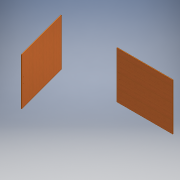
# Autodesk Inventor part: puerta_inf
Saved by Autodesk Inventor 2016 (Build 200138000, 138)
## iProperties
Created: 2015-11-25
Part Number: puerta_inf
Material: Generic
Document SubType Name: Modeling
Designer: Daniela
Density: 1 g/cm^3
Appearance: Glossy - Black
Author: Daniela
Autodesk Inventor part; units mm, degrees
ref_plane "YZ Plane" through (0, 0, 0) normal (1, 0, 0) x (0, 1, 0)
ref_plane "XZ Plane" through (0, 0, 0) normal (0, 1, 0) x (-1, 0, 0)
ref_plane "XY Plane" through (0, 0, 0) normal (0, 0, 1) x (1, 0, 0)
sketch "Sketch1" plane through (0, 0, 0) normal (0, 1, 0) x (-1, 0, 0)
  line L0 (0, 0) -> (-721.6667, 0)
  line L1 (-721.6667, 0) -> (-721.6667, 820)
  line L2 (-721.6667, 820) -> (0, 820)
  line L3 (0, 820) -> (0, 0)
  line L4 (0, 410) -> (-41, 410)
  line L5 (-41, 410) -> (-41, 460)
  line L6 (-41, 460) -> (-41, 360)
  circle A0 centre (-41, 460) radius 3
  circle A1 centre (-41, 360) radius 3
  dimension "ancho_m" = 721.6667
  dimension "h_inf" = 820
  dimension "d2" = 41
  dimension "d3" = 50
  dimension "d4" = 100
  dimension "d5" = 6
  dimension "d6" = 6
  constraints: 14 end point, 2 centre point, 2 coincident, 2 horizontal, 2 parallel, 2 perpendicular, 1 midpoint, 1 point on line
  measures "ancho_m" distance of L1.end L2.end
  measures "h_inf" distance of L0.end L1.end
  measures "d2" distance of L4.start L4.end
  measures "d3" distance of L4.end L5.end
  measures "d4" distance of L5.end L6.end
  measures "d5" diameter of A0
  measures "d6" diameter of A1
extrude "Extrusion1" add sketch "Sketch1" along normal blind 10
sketch "Boceto10" plane through (0, 0, 820) normal (0, 0, 1) x (1, 0, 0)
  line L0 (721.6667, 10) -> (0, 10) projected
  line L1 (0, 10) -> (-721.6667, 10)
  line L2 (-721.6667, 10) -> (-534.8856, -687.0765)
  line L3 (-721.6667, 10) -> (0, 10) construction
  line L4 (-534.8856, -687.0765) -> (-544.5448, -689.6647)
  line L5 (-544.5448, -689.6647) -> (-731.3259, 7.4118)
  line L6 (-731.3259, 7.4118) -> (-721.6667, 10)
  point P0 (0, 0)
  dimension "d49" = 721.6667
  dimension "d50" = 721.6667
  dimension "angulo" = 75
  dimension "d52" = 10
  dimension "d53" = 721.6667
  constraints: 12 end point, 2 horizontal, 2 perpendicular, 1 equal length
  measures "d49" distance of L0.end L1.end
  measures "d50" distance of L1.end L2.end
  measures "angulo" angle of L2 L3
  measures "d52" distance of L2.end L4.end
  measures "d53" distance of L4.end L5.end
extrude "Extrusión10" add sketch "Boceto10" against normal blind 820
sketch "Boceto11" plane through (-534.8856, -687.0765, 820) normal (0.9659258, 0.258819, 0) x (0, 0, -1)
  line L0 (0, 721.6667) -> (0, 0) projected
  line L1 (0, 0) -> (820, 0) projected
  line L2 (820, 721.6667) -> (820, 0) projected
  line L3 (0, 721.6667) -> (820, 721.6667) projected
  line L4 (0, 0) -> (820, 0) projected
  line L5 (410, 0) -> (410, 41)
  line L6 (410, 41) -> (360, 41)
  line L7 (360, 41) -> (460, 41)
  circle A0 centre (360, 41) radius 3
  circle A1 centre (460, 41) radius 3
  point P0 (820, 525.2263)
  dimension "d56" = 41
  dimension "d57" = 50
  dimension "d58" = 100
  dimension "d59" = 6
  dimension "d60" = 6
  constraints: 6 end point, 2 centre point, 2 coincident, 1 midpoint, 1 perpendicular, 1 point on line, 1 vertical
  measures "d56" distance of L5.start L5.end
  measures "d57" distance of L5.end L6.end
  measures "d58" distance of L6.end L7.end
  measures "d59" diameter of A0
  measures "d60" diameter of A1
extrude "Extrusión11" cut sketch "Boceto11" against normal up to next contours A0 | A1
equation "\"d2\" = 0.05 * h_inf"
equation "\"d49\" = ancho_m"
equation "\"d50\" = ancho_m"
equation "\"d52\" = espesor"
equation "\"d53\" = ancho_m"
equation "\"d54\" = h_inf"
equation "\"d56\" = 0.05 * h_inf"
equation "\"d61\" = h_inf"
equation "\"espesor\" = 10"
body "Solid1"
